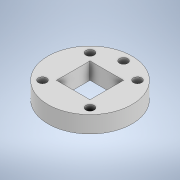
# Autodesk Inventor part: base
Saved by Autodesk Inventor 2022.3 (Build 263350000, 350)
## iProperties
Created: 2023-06-16
Part Number: base
Material: Generic
Document SubType Name: Modeling
Designer: crist
Density: 1 g/cm^3
Appearance: Default
Author: crist
Autodesk Inventor part; units mm, degrees
ref_plane "YZ Plane" through (0, 0, 0) normal (1, 0, 0) x (0, 1, 0)
ref_plane "XZ Plane" through (0, 0, 0) normal (0, 1, 0) x (-1, 0, 0)
ref_plane "XY Plane" through (0, 0, 0) normal (0, 0, 1) x (1, 0, 0)
sketch "Sketch1" plane through (0, 0, 0) normal (0, 1, 0) x (-1, 0, 0)
  circle A0 centre (-14.1421, -14.1421) radius 2.5
  circle A1 centre (-14.1421, 14.1421) radius 2.5
  line L0 (0, 0) -> (-14.1421, 14.1421)
  line L1 (0, 0) -> (0, -20)
  line L2 (0, 0) -> (-14.1421, -14.1421)
  circle A2 centre (0, -20) radius 2.5
  circle A3 centre (0, 0) radius 25
  line L3 (0, 0) -> (14.1421, 14.1421)
  line L4 (0, 0) -> (14.1421, -14.1421)
  circle A4 centre (14.1421, 14.1421) radius 2.5
  circle A5 centre (14.1421, -14.1421) radius 2.5
  line L5 (-10, 10) -> (10, 10)
  line L6 (10, 10) -> (10, -10)
  line L7 (10, -10) -> (-10, -10)
  line L8 (-10, -10) -> (-10, 10)
  line L9 (-10, 10) -> (10, -10) construction
  line L10 (10, 10) -> (-10, -10) construction
  dimension "d0" = 20
  dimension "d1" = 20
  dimension "d2" = 135
  dimension "d3" = 5
  dimension "d4" = 5
  dimension "d5" = 20
  dimension "d6" = 90
  dimension "d7" = 5
  dimension "d8" = 20
  dimension "d9" = 90
  dimension "d10" = 5
  dimension "d11" = 20
  dimension "d12" = 90
  dimension "d13" = 5
  dimension "d14" = 20
  dimension "d15" = 20
  constraints: 22 end point, 6 centre point, 6 coincident, 2 midpoint, 2 parallel, 1 horizontal, 1 perpendicular, 1 vertical
  measures "d0" distance of L0.start L1.end
  measures "d1" distance of L0.start L0.end
  measures "d2" angle of L0 L1
  measures "d3" diameter of A2
  measures "d4" diameter of A1
  measures "d5" distance of L0.start L3.end
  measures "d6" angle of L0 L3
  measures "d7" diameter of A4
  measures "d8" distance of L0.start L4.end
  measures "d9" angle of L3 L4
  measures "d10" diameter of A5
  measures "d11" distance of L0.start L2.end
  measures "d12" angle of L2 L4
  measures "d13" diameter of A0
  measures "d14" distance of L6.end L7.end
  measures "d15" distance of L5.end L6.end
extrude "Extrusion1" add sketch "Sketch1" along normal blind 10
body "Solid1"
